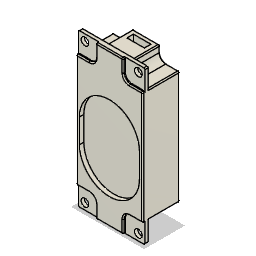
Tile (Autodesk Fusion 360 archive; units mm, degrees)
design "Speaker"
Autodesk Fusion 360 part; units mm, degrees
sketch "Sketch1" plane through (0, 0, 0) normal (0, 0, 1) x (1, 0, 0)
  line L0 (0, 0) -> (30.5, 0)
  line L1 (30.5, 0) -> (30.5, 70)
  line L2 (30.5, 70) -> (0, 70)
  line L3 (0, 70) -> (0, 0)
  line L4 (0, 35) -> (30.5, 35) construction
  line L5 (15.25, 70) -> (15.25, 0) construction
  line L6 (0, 0) -> (9, 0)
  line L7 (9, 0) -> (9, 6)
  line L8 (6, 9) -> (0, 9)
  line L9 (0, 9) -> (0, 0)
  arc A0 (9, 6) -> (6, 9) centre (6, 6) ccw
  line L10 (21.5, 0) -> (21.5, 6)
  arc A1 (24.5, 9) -> (21.5, 6) centre (24.5, 6) ccw
  line L11 (24.5, 9) -> (30.5, 9)
  line L12 (9, 70) -> (9, 64)
  arc A2 (6, 61) -> (9, 64) centre (6, 64) ccw
  line L13 (6, 61) -> (0, 61)
  line L14 (21.5, 70) -> (21.5, 64)
  arc A3 (21.5, 64) -> (24.5, 61) centre (24.5, 64) ccw
  line L15 (24.5, 61) -> (30.5, 61)
  point P0 (15.25, 35)
  dimension "d1" = 70
  dimension "d2" = 30.5
  dimension "d3" = 15.25
  dimension "d4" = 35
  dimension "d5" = 9
  dimension "d6" = 9
  dimension "d7" = 3
  constraint horizontal L0
  constraint vertical L1
  constraint horizontal L2
  constraint vertical L3
  constraint midpoint L3 L4.start
  constraint midpoint L1 L4.end
  constraint midpoint L2 L5.start
  constraint midpoint L0 L5.end
  constraint midpoint L4 P0
  constraint horizontal L6
  constraint vertical L7
  constraint horizontal L8
  constraint vertical L9
  constraint tangent L8 A0
  constraint tangent L7 A0
  constraint symmetric L5 L6.end L10.start
  constraint symmetric L5 L8.end L11.end
  constraint symmetric L5 L8.start A1.start
  constraint symmetric L5 L7.end L10.end
  constraint symmetric L5 A0 A1
  constraint symmetric L4 L6.end L12.start
  constraint symmetric L4 L8.end L13.end
  constraint symmetric L4 L8.start A2.start
  constraint symmetric L4 L7.end L12.end
  constraint symmetric L4 A0 A2
  constraint symmetric L4 L10.start L14.start
  constraint symmetric L4 L10.end L14.end
  constraint symmetric L4 A1.start A3.end
  constraint symmetric L4 A1 A3
  constraint symmetric L4 L11.end L15.end
  measures "d1" distance of L0.end L1.end
  measures "d2" distance of L0.start L0.end
  measures "d3" horizontal distance of L0.start P0
  measures "d4" vertical distance of L0.start P0
  measures "d5" distance of L7 L9
  measures "d6" distance of L0 L8
  measures "d7" radius of A0
extrude "Extrude1" add sketch "Sketch1" along normal blind 17 contours L0 L1 L2 L3 L7 L8 A0 L10 A1 L11 L12 A2 L13 L14 A3 L15
ref_plane "WorkPlane1" through (15.25, 35, 16) normal (0, 0, 1) x (1, 0, 0)
sketch "Sketch2" plane through (15.25, 35, 16) normal (0, 0, 1) x (1, 0, 0)
  line L0 (15.25, 35) -> (-15.25, 35)
  line L1 (-15.25, 35) -> (-15.25, -35)
  line L2 (-15.25, -35) -> (15.25, -35)
  line L3 (15.25, -35) -> (15.25, 35)
  line L4 (15.25, 35) -> (-15.25, -35) construction
  line L5 (-15.25, 35) -> (15.25, -35) construction
  circle A0 centre (-12.25, 32) radius 1.75
  line L6 (0, 35) -> (0, -35) construction
  line L7 (-15.25, 0) -> (15.25, 0) construction
  circle A1 centre (12.25, 32) radius 1.75
  circle A2 centre (-12.25, -32) radius 1.75
  circle A3 centre (12.25, -32) radius 1.75
  dimension "d13" = 30.5
  dimension "d14" = 70
  dimension "d33" = 3.5
  dimension "d34" = 12.25
  dimension "d35" = 32
  constraint horizontal L0
  constraint perpendicular L0 L1
  constraint parallel L0 L2
  constraint parallel L1 L3
  constraint coincident L4 origin
  constraint coincident L5 origin
  constraint midpoint L0 L6.start
  constraint midpoint L2 L6.end
  constraint midpoint L1 L7.start
  constraint midpoint L3 L7.end
  constraint symmetric A0 L6 A1
  constraint symmetric A0 L7 A2
  constraint symmetric L7 A1 A3
  measures "d13" distance of L0.start L0.end
  measures "d14" distance of L0.start L2.end
  measures "d33" diameter of A0
  measures "d34" distance of A0.centre L6
  measures "d35" distance of A0.centre L7
extrude "Extrude2" add sketch "Sketch2" against normal blind 1.5
sketch "Sketch4" plane through (0, 0, 0) normal (0, 0, -1) x (-1, 0, 0)
  line L0 (-9, 70) -> (-21.5, 70)
  line L1 (-21.5, 70) -> (-21.5, 64)
  arc A0 (-24.5, 61) -> (-21.5, 64) centre (-24.5, 64) ccw
  line L2 (-24.5, 61) -> (-30.5, 61)
  line L3 (-30.5, 61) -> (-30.5, 9)
  line L4 (-30.5, 9) -> (-24.5, 9)
  arc A1 (-21.5, 6) -> (-24.5, 9) centre (-24.5, 6) ccw
  line L5 (-21.5, 6) -> (-21.5, 0)
  line L6 (-21.5, 0) -> (-9, 0)
  line L7 (-9, 0) -> (-9, 6)
  arc A2 (-6, 9) -> (-9, 6) centre (-6, 6) ccw
  line L8 (-6, 9) -> (0, 9)
  line L9 (0, 9) -> (0, 61)
  line L10 (0, 61) -> (-6, 61)
  arc A3 (-9, 64) -> (-6, 61) centre (-6, 64) ccw
  line L11 (-9, 64) -> (-9, 70)
  line L12 (-21.5, 70) -> (-9, 70)
  line L13 (-9, 70) -> (-9, 67)
  line L14 (-9, 67) -> (-21.5, 67)
  line L15 (-21.5, 67) -> (-21.5, 70)
  line L16 (-21.5, 0) -> (-9, 0)
  line L17 (-9, 0) -> (-9, 2)
  line L18 (-9, 2) -> (-21.5, 2)
  line L19 (-21.5, 2) -> (-21.5, 0)
  dimension "d19" = 3
  dimension "d20" = 12.5
  dimension "d21" = 2
  constraint horizontal L12
  constraint vertical L13
  constraint horizontal L14
  constraint vertical L15
  constraint coincident L0.end L1.start
  constraint horizontal L16
  constraint vertical L17
  constraint horizontal L18
  constraint vertical L19
  constraint coincident L5.end L6.start
  measures "d19" distance of L0.end L14.end
  measures "d20" distance of L5.end L6.end
  measures "d21" distance of L5.end L18.end
extrude "Extrude3" cut sketch "Sketch4" against normal up to surface (14.5 mm away) contours L0 L1 L11 L12 L13 L14 L15 | L5 L6 L7 L16 L17 L18 L19
sketch "Sketch5" plane through (0, 0, 17) normal (0, 0, 1) x (1, 0, 0)
  line L0 (21.5, 70) -> (9, 70)
  line L1 (9, 70) -> (9, 64)
  arc A0 (6, 61) -> (9, 64) centre (6, 64) ccw
  line L2 (6, 61) -> (0, 61)
  line L3 (0, 61) -> (0, 9)
  line L4 (0, 9) -> (6, 9)
  arc A1 (9, 6) -> (6, 9) centre (6, 6) ccw
  line L5 (9, 6) -> (9, 0)
  line L6 (9, 0) -> (21.5, 0)
  line L7 (21.5, 0) -> (21.5, 6)
  arc A2 (24.5, 9) -> (21.5, 6) centre (24.5, 6) ccw
  line L8 (24.5, 9) -> (30.5, 9)
  line L9 (30.5, 9) -> (30.5, 61)
  line L10 (30.5, 61) -> (24.5, 61)
  arc A3 (21.5, 64) -> (24.5, 61) centre (24.5, 64) ccw
  line L11 (21.5, 64) -> (21.5, 70)
  line L12 (29, 25.75) -> (29, 36.75)
  arc A4 (29, 36.75) -> (1.5, 36.75) centre (15.25, 36.75) ccw
  line L13 (1.5, 36.75) -> (1.5, 25.75)
  arc A5 (1.5, 25.75) -> (29, 25.75) centre (15.25, 25.75) ccw
  line L14 (15.25, 25.75) -> (15.25, 36.75) construction
  dimension "d27" = 27.5
  dimension "d28" = 11
  dimension "d29" = 25.75
  dimension "d30" = 15.25
  constraint tangent L12 A4
  constraint tangent A4 L13
  constraint parallel L12 L13
  constraint tangent L13 A5
  constraint tangent L12 A5
  constraint vertical L14
  measures "d27" distance of L12 L13
  measures "d28" distance of A5.centre A4.centre
  measures "d29" distance of L6 A5.centre
  measures "d30" distance of L3 L14
extrude "Extrude4" cut sketch "Sketch5" against normal blind 2 contours L12 A4 L13 A5
sketch "Sketch6" plane through (0, 67, 0) normal (0, 1, 0) x (-1, 0, 0)
  line L0 (-9, 14.5) -> (-21.5, 14.5)
  line L1 (-21.5, 14.5) -> (-21.5, 0)
  line L2 (-21.5, 0) -> (-9, 0)
  line L3 (-9, 0) -> (-9, 14.5)
  line L4 (-11.25, 5) -> (-19.25, 5)
  line L5 (-19.25, 5) -> (-19.25, 2)
  line L6 (-19.25, 2) -> (-11.25, 2)
  line L7 (-11.25, 2) -> (-11.25, 5)
  line L8 (-11.25, 5) -> (-19.25, 2) construction
  line L9 (-19.25, 5) -> (-11.25, 2) construction
  point P0 (-15.25, 3.5)
  dimension "d39" = 3
  dimension "d40" = 8
  dimension "d41" = 2
  dimension "d43" = 15.25
  constraint horizontal L4
  constraint perpendicular L4 L5
  constraint parallel L4 L6
  constraint parallel L5 L7
  constraint coincident L8 P0
  constraint coincident L9 P0
  measures "d39" distance of L4.start L6.end
  measures "d40" distance of L4.start L4.end
  measures "d41" distance of L2 L6
  measures "d43" horizontal distance of origin P0
extrude "Extrude5" cut sketch "Sketch6" against normal blind 10 contours L4 L5 L6 L7
fillet "Fillet3" radius 0.5 4 edges at (30.5, 70, 15.25) (0, 70, 15.25) (0, 0, 15.25) (30.5, 0, 15.25)
fillet "Fillet3" radius 0.5 16 edges at (0, 9, 7.25) (0, 9, 16.5) (9, 0, 16.5) (9, 2, 7.25) (21.5, 2, 7.25) (21.5, 0, 16.5) (30.5, 9, 16.5) (30.5, 9, 7.25) (30.5, 61, 16.5) (30.5, 61, 7.25) (21.5, 67, 7.25) (21.5, 70, 16.5) (9, 70, 16.5) (9, 67, 7.25) (0, 61, 7.25) (0, 61, 16.5)
fillet "Fillet3" radius 0.5 16 edges at (27.5, 61, 17) (22.3787, 61.8787, 17) (21.5, 67, 17) (9, 67, 17) (8.1213, 61.8787, 17) (3, 61, 17) (15.25, 70, 17) (0, 35, 17) (3, 9, 17) (8.1213, 8.1213, 17) (9, 3, 17) (15.25, 0, 17) (21.5, 3, 17) (22.3787, 8.1213, 17) (27.5, 9, 17) (30.5, 35, 17) 1 faces at (18.0516, 43.7072, 0)
equation "d28 = 38.5 mm - 27.5 mm"
equation "d29 = 12 mm + ( ( 27.5 / 2 ) * 1 mm )"
equation "d30 = ( 30.5 / 2 ) * 1 mm"
equation "d34 = ( ( 21 + 3.5 ) / 2 ) * 1 mm"
equation "d35 = ( ( 60.5 + 3.5 ) / 2 ) * 1 mm"
equation "d43 = ( 30.5 / 2 ) * 1 mm"
